Autodesk Inventor part; units mm, degrees
(part 2 of 2)
  spline S29 degree 5 poles (-11.4815, 297.1367) (-11.2868, 297.7078) (-11.054, 298.2658) (-10.7757, 298.8036) (-10.1641, 299.6273) (-9.2825, 300.1216) (-8.8967, 300.242) (-8.2268, 300.3042) (-7.5704, 300.1886) (-7.3067, 300.1162) (-6.8416, 299.9427) (-6.4152, 299.6885) (-6.2327, 299.5593) (-5.9151, 299.2923) (-5.6399, 298.9827) (-5.5227, 298.8316) (-5.3216, 298.535) (-5.1569, 298.2169) (-5.088, 298.0645) (-4.9725, 297.7683) (-4.8861, 297.4624) (-4.8517, 297.3156) (-4.7977, 297.0284) (-4.768, 296.7376) (-4.7593, 296.5963) (-4.7532, 296.3148) (-4.7685, 296.0336) (-4.7812, 295.8942) (-4.8161, 295.6137) (-4.8678, 295.3358) (-4.8978, 295.1962) (-4.9654, 294.9139) (-5.0452, 294.6348) (-5.0885, 294.4937) (-5.1817, 294.2079) (-5.2855, 293.9258) (-5.3411, 293.7832) (-5.461, 293.4952) (-5.597, 293.2145) (-5.6711, 293.0739) (-5.8352, 292.793) (-6.0304, 292.5327) (-6.1396, 292.4067) (-6.3814, 292.1712) (-6.6618, 291.9834) (-6.8129, 291.9029) (-7.1268, 291.7743) (-7.4592, 291.7066) (-7.6266, 291.6879) (-7.9605, 291.6768) (-8.2927, 291.7127) (-8.4562, 291.7409) (-8.7799, 291.8165) (-9.0932, 291.9277) (-9.2471, 291.9916) (-9.5485, 292.1357) (-9.8333, 292.3101) (-9.9715, 292.405) (-10.2373, 292.6091) (-10.4799, 292.8405) (-10.5948, 292.9627) (-10.803, 293.21) (-10.9841, 293.4777) (-11.0647, 293.6109) (-11.1386, 293.7478) (-11.2057, 293.8879) knots 0 0 0 0 0 0 0.143413 0.143413 0.143413 0.23652 0.23652 0.23652 0.30109 0.30109 0.30109 0.354053 0.354053 0.354053 0.399372 0.399372 0.399372 0.43907 0.43907 0.43907 0.474852 0.474852 0.474852 0.508487 0.508487 0.508487 0.541736 0.541736 0.541736 0.575659 0.575659 0.575659 0.610726 0.610726 0.610726 0.647109 0.647109 0.647109 0.684848 0.684848 0.684848 0.724326 0.724326 0.724326 0.76474 0.76474 0.76474 0.804598 0.804598 0.804598 0.84396 0.84396 0.84396 0.8835 0.8835 0.8835 0.923261 0.923261 0.923261 0.963062 0.963062 0.963062 1 1 1 1 1 1
  point P0 (0, 0)
  point P1 (7.3159, 313.8693)
  point P2 (7.3159, 312.4495)
  point P3 (7.2094, 311.1717)
  point P4 (8.2819, 310.9976)
  point P5 (9.4375, 310.9976)
  point P6 (10.0795, 311.2643)
  point P7 (10.4647, 312.2619)
  point P8 (10.6129, 313.4076)
  point P9 (10.6919, 314.2472)
  point P10 (10.9152, 315.2286)
  point P11 (10.9152, 316.1226)
  point P12 (9.9942, 316.4097)
  point P13 (9.2676, 316.4572)
  point P14 (8.7718, 316.4097)
  point P15 (3.9875, 303.786)
  point P16 (2.8022, 302.8701)
  point P17 (1.7247, 301.0921)
  point P18 (1.1277, 298.3868)
  point P19 (2.5467, 293.0044)
  point P20 (9.0521, 293.9802)
  point P21 (10.5722, 296.9628)
  point P22 (10.7945, 299.3941)
  point P23 (10.1276, 302.2422)
  point P24 (9.1313, 303.7964)
  point P25 (3.9561, 298.3879)
  point P26 (0.5117, 298.9476)
  point P27 (-7.3084, 295.8675)
  constraints: 70 parallel, 60 end point, 32 point on circle, 13 centre point, 11 perpendicular, 7 point on line, 2 horizontal, 1 midpoint, 142 other
equation "\"d0\" = 0.5 * PortalBreite"
equation "\"d1\" = 0.5 * PortalBreite"
equation "\"d25\" = Durchmesser"
equation "\"d26\" = d24"
equation "\"d27\" = d23"
equation "\"d30\" = Durchmesser"
equation "\"d31\" = Durchmesser"
equation "\"d32\" = d24"
equation "\"d33\" = d24"
equation "\"d35\" = d34"
equation "\"d46\" = d47"
equation "\"d48\" = d45"
equation "\"d8\" = Stärke"
equation "\"d3\" = PortalHoehe"
equation "\"d6\" = GesammtHoehe"
equation "\"PortalBreite\" = 163"
equation "\"Biegeradius\" = Stärke"
equation "\"BreiteBiegungsfreistellung\" = Stärke"
equation "\"TiefeBiegungsfreistellung\" = 0.5 * Stärke"
equation "\"GrößeEckenfreistellung\" = 4 * Stärke"
equation "\"MinimalRest\" = 2 * Stärke"
equation "\"Übergangsradius\" = Biegeradius"
equation "\"JacobiRadiusGröße\" = Biegeradius"
equation "\"Abstandsgröße\" = Stärke"
equation "\"Stärke\" = 2"
